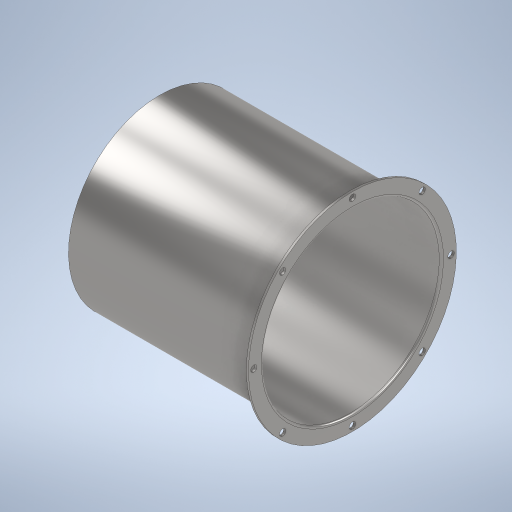
# Autodesk Inventor part: outerwall part 1
Saved by Autodesk Inventor 2023 (Build 270158000, 158)
## iProperties
Created: 2022-07-20
Part Number: outerwall part 1
Material: Stainless Steel
Document SubType Name: Modeling
Designer: station
Density: 8 g/cm^3
Appearance: Semi-Polished
Author: station
Autodesk Inventor part; units mm, degrees
ref_plane "YZ Plane" through (0, 0, 0) normal (1, 0, 0) x (0, 1, 0)
ref_plane "XZ Plane" through (0, 0, 0) normal (0, 1, 0) x (-1, 0, 0)
ref_plane "XY Plane" through (0, 0, 0) normal (0, 0, 1) x (1, 0, 0)
sketch "Sketch1" plane through (0, 0, 0) normal (0, 0, 1) x (1, 0, 0)
  arc A0 (180.1312, 21.4516) -> (182.1847, 21.7676) centre (180.1312, 28.2803) ccw
  arc A1 (166.724, 25.044) -> (180.1312, 21.4516) centre (180.1312, 48.266) ccw
  line L0 (123.3912, 50.0622) -> (166.724, 25.044)
  arc A2 (123.3912, 50.0622) -> (30.0219, 75.0805) centre (30.0219, -111.6581) ccw
  line L1 (0, 75.0805) -> (30.0219, 75.0805)
  line L2 (0, 3.5755) -> (319.1694, 3.5755)
  line L3 (182.1847, 21.7676) -> (237.115, 39.0871)
  line L4 (0, 86.6805) -> (30.0219, 86.6805)
  line L5 (180.1312, 33.0516) -> (237.115, 51.0185)
  line L6 (180.1312, 33.0516) -> (239.8803, 33.0516) construction
  line L7 (0, 88.6805) -> (30.0219, 88.6805)
  line L8 (236.5136, 52.9259) -> (180.1312, 35.1486)
  line L9 (237.115, 39.0871) -> (237.115, 127.9105) construction
  line L10 (237.115, 51.0185) -> (236.5136, 52.9259)
  line L11 (0, 86.6805) -> (0, 88.6805)
  line L12 (180.1312, 33.0516) -> (180.1312, 35.1486)
  line L13 (180.1312, 33.0516) -> (180.1312, -12.2002)
  line L14 (30.0219, 88.6805) -> (176.1312, 88.6805)
  line L15 (30.0219, 86.6805) -> (178.1312, 86.6805)
  line L16 (180.1312, 88.6805) -> (180.1312, 100.6805)
  line L17 (178.1312, 90.6805) -> (178.1312, 100.6805)
  line L18 (178.1312, 100.6805) -> (180.1312, 100.6805)
  arc A3 (178.1312, 86.6805) -> (180.1312, 88.6805) centre (178.1312, 88.6805) ccw
  arc A4 (176.1312, 88.6805) -> (178.1312, 90.6805) centre (176.1312, 90.6805) ccw
  point P0 (0, 0)
  point P1 (180.1312, 86.6805)
  dimension "d0" = 30.0219
  dimension "d1" = 186.7386
  dimension "d2" = 0
  dimension "d3" = 0
  dimension "d4" = 71.505
  dimension "d10" = 17.5
  dimension "d11" = 54.9303
  dimension "d13" = 11.6
  dimension "d19" = 17.5
  dimension "d20" = 2
  dimension "d31" = 14
  dimension "d32" = 2
  dimension "d33" = 2
  constraints: 38 end point, 10 point on circle, 5 centre point, 4 horizontal, 4 tangent, 4 vertical, 3 parallel, 2 point on line, 1 equal length, 1 equal radius, 1 perpendicular
  measures "d0" distance of L1.start L1.end
  measures "d1" radius of A2
  measures "d2" distance of A2.end L1.end
  measures "d3" distance of L0.start A2.start
  measures "d4" distance between parallel lines of L2 L1
  measures "d10" angle of L2 L3
  measures "d11" horizontal distance of L3.start L3.end
  measures "d13" distance between parallel lines of L1 L4
  measures "d19" angle of L6 L5
  measures "d20" distance between parallel lines of L4 L7
  measures "d31" distance of point (180.131, 86.68) L16.end
  measures "d32" distance between parallel lines of L16 L17
  measures "d33" radius of A3
revolve "Revolution3" add sketch "Sketch1" angle 360 about axis through (0, 3.5755, 0) along (1, 0, 0) contours L11 L7 L14 A4 L17 L18 L16 A3 L15 L4
sketch "Sketch2" plane through (180.1312, 3.5755, 0) normal (1, 0, 0) x (0, 0, -1)
  circle A0 centre (0, 0) radius 97.105 projected
  line L0 (0, 97.105) -> (0, 85.105) construction
  circle A1 centre (0, 0) radius 85.105 projected
  line L1 (0, 97.105) -> (0, 92.105)
  circle A2 centre (0, 92.105) radius 3
  point P0 (0, -3.5755)
  dimension "d35" = 5
  dimension "d36" = 6
  constraints: 4 end point, 2 vertical alignment, 1 centre point, 1 coincident, 1 point on line, 1 vertical, 2 other
  measures "d35" distance of L0.start L1.end
  measures "d36" diameter of A2
extrude "Extrusion1" cut sketch "Sketch2" against normal blind 2 contours A2
pattern_circular "Circular Pattern1" count 8 over 360 about axis through (179.1312, 3.5755, 0) along (1, 0, 0) of "Extrusion1"
body "Solid3"
